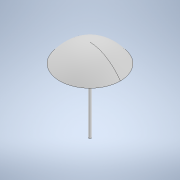
# Autodesk Inventor part: knitHatHolder
Saved by Autodesk Inventor 2021 (Build 250183000, 183)
## iProperties
Created: 2020-11-14
Part Number: knitHatHolder
Material: Generic
Document SubType Name: Modeling
Designer: jjaken
Density: 1 g/cm^3
Appearance: Default
Author: jjaken
Autodesk Inventor part; units mm, degrees
ref_plane "YZ Plane" through (0, 0, 0) normal (1, 0, 0) x (0, 1, 0)
ref_plane "XZ Plane" through (0, 0, 0) normal (0, 1, 0) x (-1, 0, 0)
ref_plane "XY Plane" through (0, 0, 0) normal (0, 0, 1) x (1, 0, 0)
sketch "Sketch1" plane through (0, 0, 0) normal (0, 0, 1) x (1, 0, 0)
  ellipse E0 centre (0, 0) end of major axis (133.35, 0) minor radius 228.6 (133.35, 0) -> (0, 228.6) ccw
  line L0 (0, 0) -> (133.35, 0)
  line L1 (0, 228.6) -> (0, 0)
  dimension "d0" = 228.6
  dimension "d1" = 133.35
  constraints: 4 end point, 1 coincident, 1 horizontal, 1 perpendicular, 4 other
revolve "Revolution1" add sketch "Sketch1" angle 360 about axis through (0, 228.6, 0) along (0, -1, 0)
shell "Shell1" thickness 3 removed faces 1 at (11.9667, 0, 37.766)
sketch "Sketch3" plane through (0, 0, 0) normal (0, -1, 0) x (1, 0, 0)
  line L0 (180.2464, 153.6445) -> (-162.3461, 153.6445)
  line L1 (-162.3461, 153.6445) -> (-162.3461, -158.1196)
  line L2 (-162.3461, -158.1196) -> (180.2464, -158.1196)
  line L3 (180.2464, -158.1196) -> (180.2464, 153.6445)
  point P0 (0, 0)
  constraints: 8 end point, 2 parallel, 1 horizontal, 1 perpendicular
extrude "Extrusion2" cut sketch "Sketch3" against normal blind 177.8
sketch "Sketch2" plane through (0, 0, 0) normal (0, -1, 0) x (1, 0, 0)
  line L0 (133.35, 0) -> (0, 0) projected
  circle A0 centre (0, 0) radius 3
  dimension "d4" = 6
  constraints: 1 centre point, 1 coincident
  measures "d4" diameter of A0
extrude "Extrusion1" add sketch "Sketch2" against normal up to next
body "Solid1"
